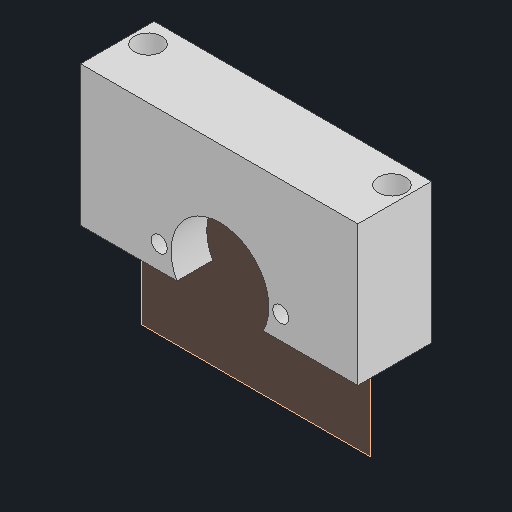
# Autodesk Inventor part: right_motor_floor
Saved by Autodesk Inventor 2023 (Build 270158000, 158)
## iProperties
Created: 2024-04-14
Part Number: right_motor_floor
Material: Generic
Document SubType Name: Modeling
Designer: szymo
Density: 1 g/cm^3
Appearance: Default
Author: szymo
Autodesk Inventor part; units mm, degrees
ref_plane "YZ Plane" through (0, 0, 0) normal (1, 0, 0) x (0, 1, 0)
ref_plane "Work Plane1" through (0, 0, 0) normal (0, 0, 1) x (1, 0, 0)
sketch "Sketch1" plane through (0, 0, 0) normal (0, 0, 1) x (1, 0, 0)
  circle A0 centre (8, 0) radius 1.0564 projected
  circle A1 centre (-8, 0) radius 1.0564 projected
  circle A2 centre (0, 0) radius 5 projected
  circle A3 centre (0, 0) radius 13.7 projected
  line L0 (-18.375, 15.375) -> (-18.375, 1) projected
  line L1 (-18.375, 1) -> (-13.6635, 1) projected
  arc A4 (13.6635, 1) -> (-13.6635, 1) centre (0, 0) ccw projected
  line L2 (13.6635, 1) -> (18.1635, 1) projected
  line L3 (18.1635, 1) -> (18.1635, 15.375) projected
  line L4 (18.1635, 15.375) -> (-18.375, 15.375) projected
  line L5 (18.1635, 15.375) -> (-18.375, 15.375)
  line L6 (-18.375, 15.375) -> (-18.375, -3.0565)
  line L7 (-18.375, -3.0565) -> (18.1635, -3.0565)
  line L8 (18.1635, -3.0565) -> (18.1635, 15.375)
  line L9 (18.1635, -5.0565) -> (12.7327, -5.0565) projected
  circle A5 centre (0, 0) radius 6.4423
  arc A6 (2.7565, 5.1523) -> (1.2674, 3.6504) centre (5.3281, 1.1135) ccw projected
  arc A7 (1.2674, 3.6504) -> (0.6807, 3.8037) centre (0, 0) ccw projected
  arc A8 (0.6807, 3.8037) -> (0.1169, 5.8421) centre (-4.102, 3.578) ccw projected
  arc A9 (0.1169, 5.8421) -> (-0.7984, 5.7885) centre (0, 0) ccw projected
  arc A10 (-0.7984, 5.7885) -> (-1.1203, 3.6981) centre (3.6561, 4.0326) ccw projected
  arc A11 (-1.1203, 3.6981) -> (-1.685, 3.4774) centre (0, 0) ccw projected
  arc A12 (-1.685, 3.4774) -> (-3.3393, 4.7951) centre (-5.4217, 0.4836) ccw projected
  arc A13 (-3.3393, 4.7951) -> (-4.0483, 4.2137) centre (0, 0) ccw projected
  arc A14 (-4.0483, 4.2137) -> (-3.0801, 2.3334) centre (0.5875, 5.4114) ccw projected
  arc A15 (-3.0801, 2.3334) -> (-3.4072, 1.8228) centre (0, 0) ccw projected
  arc A16 (-3.4072, 1.8228) -> (-5.52, 1.9165) centre (-4.6705, -2.7956) ccw projected
  arc A17 (-5.52, 1.9165) -> (-5.7519, 1.0294) centre (0, 0) ccw projected
  arc A18 (-5.7519, 1.0294) -> (-3.8633, 0.0773) centre (-2.7054, 4.7233) ccw projected
  arc A19 (-3.8633, 0.0773) -> (-3.8279, -0.528) centre (0, 0) ccw projected
  arc A20 (-3.8279, -0.528) -> (-5.5923, -1.6941) centre (-2.1353, -5.0069) ccw projected
  arc A21 (-5.5923, -1.6941) -> (-5.2584, -2.5481) centre (0, 0) ccw projected
  arc A22 (-5.2584, -2.5481) -> (-3.171, -2.2083) centre (-4.965, 2.231) ccw projected
  arc A23 (-3.171, -2.2083) -> (-2.7865, -2.6771) centre (0, 0) ccw projected
  arc A24 (-2.7865, -2.6771) -> (-3.5285, -4.6576) centre (1.2155, -5.3058) ccw projected
  arc A25 (-3.5285, -4.6576) -> (-2.7565, -5.1523) centre (0, 0) ccw projected
  arc A26 (-2.7565, -5.1523) -> (-1.2674, -3.6504) centre (-5.3281, -1.1135) ccw projected
  arc A27 (-1.2674, -3.6504) -> (-0.6807, -3.8037) centre (0, 0) ccw projected
  arc A28 (-0.6807, -3.8037) -> (-0.1169, -5.8421) centre (4.102, -3.578) ccw projected
  arc A29 (-0.1169, -5.8421) -> (0.7984, -5.7885) centre (0, 0) ccw projected
  arc A30 (0.7984, -5.7885) -> (1.1203, -3.6981) centre (-3.6561, -4.0326) ccw projected
  arc A31 (1.1203, -3.6981) -> (1.685, -3.4774) centre (0, 0) ccw projected
  arc A32 (1.685, -3.4774) -> (3.3393, -4.7951) centre (5.4217, -0.4836) ccw projected
  arc A33 (3.3393, -4.7951) -> (4.0483, -4.2137) centre (0, 0) ccw projected
  arc A34 (4.0483, -4.2137) -> (3.0801, -2.3334) centre (-0.5875, -5.4114) ccw projected
  arc A35 (3.0801, -2.3334) -> (3.4072, -1.8228) centre (0, 0) ccw projected
  arc A36 (3.4072, -1.8228) -> (5.52, -1.9165) centre (4.6705, 2.7956) ccw projected
  arc A37 (5.52, -1.9165) -> (5.7519, -1.0294) centre (0, 0) ccw projected
  arc A38 (5.7519, -1.0294) -> (3.8633, -0.0773) centre (2.7054, -4.7233) ccw projected
  arc A39 (3.8633, -0.0773) -> (3.8279, 0.528) centre (0, 0) ccw projected
  arc A40 (3.8279, 0.528) -> (5.5923, 1.6941) centre (2.1353, 5.0069) ccw projected
  arc A41 (5.5923, 1.6941) -> (5.2584, 2.5481) centre (0, 0) ccw projected
  arc A42 (5.2584, 2.5481) -> (3.171, 2.2083) centre (4.965, -2.231) ccw projected
  arc A43 (3.171, 2.2083) -> (2.7865, 2.6771) centre (0, 0) ccw projected
  arc A44 (2.7865, 2.6771) -> (3.5285, 4.6576) centre (-1.2155, 5.3058) ccw projected
  arc A45 (3.5285, 4.6576) -> (2.7565, 5.1523) centre (0, 0) ccw projected
  point P0 (-5.6711, -3.0565)
  point P1 (-6.9927, -0.3186)
  point P2 (-6.9927, 0.3186)
  point P3 (6.9927, 0.3186)
  point P4 (6.9927, -0.3186)
  point P5 (5.6711, -3.0565)
  point P6 (0.3418, -6.4333)
  point P7 (0.3418, -5.8333)
  dimension "d0" = 2
  dimension "d4" = 0.6
  constraints: 8 end point, 2 parallel, 1 coincident, 1 horizontal, 1 perpendicular, 1 point on circle, 3 other
  measures "d0" distance between parallel lines of L9 L7
  measures "d4" distance of point (0.342, -6.433) point (0.342, -5.833)
ref_plane "Work Plane2" through (-70.375, 15.375, 4.7) normal (0, 0, -1) x (0, 1, 0)
extrude "Extrusion1" add sketch "Sketch1" along normal up to surface (4.7 mm away) contours A5 L7 A3 | A3 L2 L8 L7 | L7 L6 L1 A3 | A3 L1 L0 L4 L3 L2 picked at (8.5523, 7.2456)
sketch "Sketch2" plane through (0, 0, 0) normal (0, 0, -1) x (-1, 0, 0)
  circle A0 centre (-8, 0) radius 1.0564 projected
  circle A1 centre (8, 0) radius 1.0564 projected
  circle A2 centre (0, 0) radius 5 projected
  circle A3 centre (0, 0) radius 13.7 projected
  line L0 (-5.6711, -3.0565) -> (-18.1635, -3.0565) projected
  arc A4 (5.6711, -3.0565) -> (-5.6711, -3.0565) centre (0, 0) ccw projected
  line L1 (18.375, -3.0565) -> (5.6711, -3.0565) projected
  line L2 (18.375, 15.375) -> (18.375, -3.0565) projected
  line L3 (-18.1635, 15.375) -> (18.375, 15.375) projected
  line L4 (-18.1635, -3.0565) -> (-18.1635, 15.375) projected
  circle A5 centre (-8, 0) radius 1.0564 projected
  circle A6 centre (8, 0) radius 1.0564 projected
  point P0 (-13.3547, -3.0565)
  point P1 (13.3547, -3.0565)
ref_plane "Work Plane3" through (-14.375, -14.375, -5) normal (0, 0, 1) x (1, 0, 0)
extrude "Extrusion2" add sketch "Sketch2" along normal up to surface (5 mm away) contours A3 L0 L4 L3 L2 L1
sketch "Sketch3" plane through (5.6711, -3.0565, 4.7) normal (0, -1, 0) x (1, 0, 0)
  circle A0 centre (10.2923, -6.7) radius 1.8 projected
  circle A1 centre (-21.8461, -6.7) radius 1.8 projected
  point P0 (-5.6711, -4.7)
  constraints: 2 coincident
hole "Hole1" at (15.9635, -3.0565, -2) at (-16.175, -3.0565, -2) direction (0, 1, 0) diameter 3.6 end through all counterbore diameter 11 counterbore depth 0 clearance for "Hex Head Cap Screw ISO 24017" size "M3" standard "ISO"
body "Solid1"
